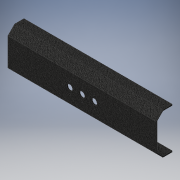
# Autodesk Inventor part: ChassisMainBracket
Saved by Autodesk Inventor 2016 (Build 200138000, 138)
## iProperties
Created: 2015-08-06
Part Number: ChassisMainBracket
Material: Generic
Document SubType Name: Modeling
Designer: lachesis
Density: 1 g/cm^3
Appearance: Black Cast
Author: lachesis
Autodesk Inventor part; units mm, degrees
note: some values were not read from the file. Chosen so that the rebuilt part matches the saved one: direction of "Hole1"; direction of "Hole2".
ref_plane "YZ Plane" through (0, 0, 0) normal (1, 0, 0) x (0, 1, 0)
ref_plane "XZ Plane" through (0, 0, 0) normal (0, 1, 0) x (-1, 0, 0)
ref_plane "XY Plane" through (0, 0, 0) normal (0, 0, 1) x (1, 0, 0)
sketch "Sketch1" plane through (0, 0, 0) normal (1, 0, 0) x (0, 1, 0)
  line L0 (18.8, 0) -> (-18.8, 0)
  line L1 (-18.8, 0) -> (-18.8, 1.6)
  line L2 (-18.8, 1.6) -> (18.8, 1.6)
  line L3 (18.8, 1.6) -> (18.8, 0)
  line L4 (18.8, 1.6) -> (28.2, -7.7473)
  line L5 (28.2, -7.7473) -> (28.2, -20.4563)
  line L6 (28.2, -20.4563) -> (26.6, -20.4563)
  line L7 (26.6, -20.4563) -> (26.6, -7.7563)
  line L8 (26.6, -7.7563) -> (18.8, 0)
  line L9 (0, 0) -> (0, 1.6)
  line L10 (-18.8, 1.6) -> (-28.2, -7.7473)
  line L11 (-28.2, -7.7473) -> (-28.2, -20.4563)
  line L12 (-26.6, -20.4563) -> (-26.6, -7.7563)
  line L13 (-26.6, -7.7563) -> (-18.8, 0)
  line L14 (-28.2, -20.4563) -> (-26.6, -20.4563)
  dimension "d0" = 1.6
  dimension "d1" = 1.6
  dimension "d3" = 11
  dimension "d4" = 12.7
  dimension "d5" = 56.4
  dimension "d8" = 7.8
  constraints: 30 end point, 4 symmetric about line, 3 parallel, 3 perpendicular, 2 horizontal, 2 midpoint, 1 coincident, 1 vertical
  measures "d0" distance between parallel lines of L2 L0
  measures "d1" distance between parallel lines of L7 L5
  measures "d3" distance of L0.start L7.end
  measures "d4" distance of L6.end L7.end
  measures "d5" distance between parallel lines of L11 L5
  measures "d8" horizontal distance of L7.end L0.start
extrude "Extrusion1" add sketch "Sketch1" along normal blind 201.549
sketch "Sketch2" plane through (0, 28.2, -7.7473) normal (0, 1, 0) x (1, 0, 0)
  line L0 (0, 12.709) -> (0, 0) projected
  line L1 (0, 0) -> (201.549, 0) projected
  line L2 (201.549, 12.709) -> (201.549, 0) projected
  line L3 (0, 12.709) -> (201.549, 12.709) projected
  point P0 (0, -7.7473)
  point P1 (5.6, 6.3545)
  point P2 (195.949, 6.3545)
  point P3 (0, 6.3545)
  point P4 (201.549, 6.3545)
  dimension "d11" = 5.6
  dimension "d12" = 5.6
  constraints: 3 horizontal alignment, 2 midpoint
  measures "d11" distance from line of L0 point (5.6, 6.354)
  measures "d12" distance from line of L2 point (195.949, 6.354)
hole "Hole1" at (5.6, 28.2, -14.1018) at (195.949, 28.2, -14.1018) direction (0, -1, 0) diameter 2.459 end up to surface
sketch "Sketch3" plane through (0, -28.2, -20.4563) normal (0, -1, 0) x (1, 0, 0)
  circle A0 centre (195.949, 6.3545) radius 1.2295 projected
  circle A1 centre (5.6, 6.3545) radius 1.2295 projected
  point P0 (0, 20.4563)
  constraints: 2 coincident
hole "Hole2" at (195.949, -28.2, -14.1018) at (5.6, -28.2, -14.1018) direction (0, 1, 0) diameter 2.459 end up to surface
sketch "Sketch4" plane through (0, -18.8, 1.6) normal (0, 0, 1) x (1, 0, 0)
  line L0 (0, 37.6) -> (0, 0) projected
  line L1 (0, 0) -> (201.549, 0) projected
  line L2 (201.549, 37.6) -> (201.549, 0) projected
  line L3 (0, 37.6) -> (201.549, 37.6) construction
  circle A0 centre (100.7745, 18.8) radius 4.0005
  circle A1 centre (100.7745, 27.1312) radius 1.1938
  circle A2 centre (92.4433, 18.8) radius 1.1938
  circle A3 centre (100.7745, 10.4688) radius 1.1938
  circle A4 centre (109.1057, 18.8) radius 1.1938
  line L4 (0, 37.6) -> (201.549, 37.6) projected
  circle A5 centre (84.1121, 18.8) radius 4.0005
  circle A6 centre (84.1121, 27.1312) radius 1.1938
  circle A7 centre (75.7809, 18.8) radius 1.1938
  circle A8 centre (84.1121, 10.4688) radius 1.1938
  circle A9 centre (92.4433, 18.8) radius 1.1938
  circle A10 centre (117.4369, 18.8) radius 4.0005
  circle A11 centre (117.4369, 27.1312) radius 1.1938
  circle A12 centre (109.1057, 18.8) radius 1.1938
  circle A13 centre (117.4369, 10.4688) radius 1.1938
  circle A14 centre (125.7681, 18.8) radius 1.1938
  point P0 (0, 18.8)
  point P1 (100.7745, 37.6)
  point P2 (201.549, 18.8)
  point P3 (100.7745, 37.6)
  dimension "d27" = 8.001
  dimension "d28" = 8.3312
  dimension "d29" = 2.3876
  dimension "d32" = 360
  dimension "d39" = 8.001
  dimension "d40" = 8.3312
  dimension "d41" = 2.3876
  dimension "d42" = 360
  dimension "d47" = 8.001
  dimension "d48" = 8.3312
  dimension "d49" = 2.3876
  dimension "d50" = 360
  dimension "d53" = 16.6624
  dimension "d54" = 16.6624
  constraints: 15 centre point, 3 midpoint, 2 coincident, 2 vertical alignment, 1 horizontal alignment, 27 other
  measures "d27" diameter of A0
  measures "d28" distance of A0.centre A1.centre
  measures "d29" diameter of A1
  measures "d39" diameter of A5
  measures "d40" distance of A5.centre A6.centre
  measures "d41" diameter of A6
  measures "d47" diameter of A10
  measures "d48" distance of A10.centre A11.centre
  measures "d49" diameter of A11
  measures "d53" distance of A3.centre A8.centre
  measures "d54" distance of A3.centre A13.centre
extrude "Extrusion2" cut sketch "Sketch4" against normal through all contours A0 | A1 | A2 | A3 | A4 | A5 | A6 | A7 | A8 | A10 | A11 | A13 | A14
equation "\"d12\" = d11"
equation "\"d54\" = d53"
body "Solid1"
